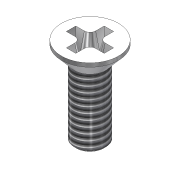
# Autodesk Inventor part: Part32
Saved by Autodesk Inventor 2011 (Build 150239000, 239)
## iProperties
Created: 2012-04-09
Part Number: Part32
Material: Steel
Document SubType Name: Modeling
Designer: jhanson2
Density: 7.85 g/cm^3
Author: jhanson2
Autodesk Inventor part; units mm, degrees
ref_plane "YZ Plane" through (0, 0, 0) normal (1, 0, 0) x (0, 1, 0)
ref_plane "XZ Plane" through (0, 0, 0) normal (0, 1, 0) x (-1, 0, 0)
ref_plane "XY Plane" through (0, 0, 0) normal (0, 0, 1) x (1, 0, 0)
sketch "Sketch1" plane through (0, 0, 0) normal (0, 0, 1) x (1, 0, 0)
  line L0 (0, 0) -> (-2.0828, 0)
  line L1 (-2.0828, 0) -> (-2.0828, 9.144)
  line L2 (-2.0828, 9.144) -> (0, 9.144)
  line L3 (0, 9.144) -> (0, 0)
  line L4 (-2.0828, 9.144) -> (-3.81, 11.176)
  line L5 (-3.81, 11.176) -> (-3.81, 11.684)
  line L6 (-3.81, 11.684) -> (0, 11.684)
  line L7 (0, 11.684) -> (0, 9.144)
  dimension "d0" = 4.1656
  dimension "d1" = 9.144
  dimension "d2" = 7.62
  dimension "d3" = 0.508
  dimension "d4" = 2.54
  constraints: 16 end point, 3 parallel, 3 perpendicular, 1 horizontal
  measures "d0" diameter of L1 L3
  measures "d1" distance of L0.end L1.end
  measures "d2" diameter of L5.end L7
  measures "d3" distance from line of L4.end L6
  measures "d4" distance between parallel lines of L2 L6
revolve "Revolution1" add sketch "Sketch1" angle 360 about axis through (0, 9.144, 0) along (0, -1, 0)
thread "Thread1" size "8-32 UNC" class "2A" standard "ANSI Unified Screw Threads" full length
sketch "Sketch2" plane through (0, 11.684, 0) normal (0, 1, 0) x (1, 0, 0)
  circle A0 centre (0, 0) radius 3.81 projected
  line L0 (2.54, 0.635) -> (2.54, -0.635)
  line L1 (-2.54, -0.635) -> (-2.54, 0.635)
  line L2 (-0.635, 2.54) -> (0.635, 2.54)
  line L3 (0.635, -2.54) -> (-0.635, -2.54)
  line L4 (-0.635, -2.54) -> (-0.635, -1.397)
  line L5 (-0.635, 1.397) -> (-0.635, 2.54)
  line L6 (2.54, -0.635) -> (1.397, -0.635)
  line L7 (-1.397, -0.635) -> (-2.54, -0.635)
  line L8 (0.635, 2.54) -> (0.635, 1.397)
  line L9 (0.635, -1.397) -> (0.635, -2.54)
  line L10 (-2.54, 0.635) -> (-1.397, 0.635)
  line L11 (1.397, 0.635) -> (2.54, 0.635)
  line L12 (0, 2.54) -> (0, 0) construction
  line L13 (0, 0) -> (-2.54, 0) construction
  arc A1 (-0.635, -1.397) -> (-1.397, -0.635) centre (-1.397, -1.397) ccw
  arc A2 (1.397, -0.635) -> (0.635, -1.397) centre (1.397, -1.397) ccw
  arc A3 (0.635, 1.397) -> (1.397, 0.635) centre (1.397, 1.397) ccw
  arc A4 (-1.397, 0.635) -> (-0.635, 1.397) centre (-1.397, 1.397) ccw
  dimension "d8" = 1.27
  dimension "d9" = 5.08
  dimension "d10" = 0.762
  constraints: 28 end point, 10 parallel, 8 point on circle, 8 tangent, 4 centre point, 4 collinear, 4 equal length, 4 horizontal, 4 perpendicular, 3 equal radius, 2 midpoint, 1 vertical
  measures "d8" distance of L2.start L2.end
  measures "d9" distance between parallel lines of L3 L2
  measures "d10" radius of A1
extrude "Extrusion1" cut sketch "Sketch2" against normal blind 2.54 draft -14 contours L0 L6 A2 L9 L3 L4 A1 L7 L1 L10 A4 L5 L2 L8 A3 L11
chamfer "Chamfer1" distance 0.254 angle 45 1 edges at (2.0828, 0, 0)
body "Solid1"
